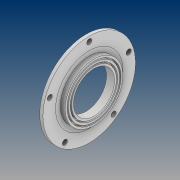
# Autodesk Inventor part: LABYRINTHOSeisodos
Saved by Autodesk Inventor 2021 (Build 250183000, 183)
## iProperties
Created: 2021-01-09
Part Number: LABYRINTHOSeisodos
Material: Generic
Document SubType Name: Modeling
Designer: Διογενης Τσιχλακης
Density: 1 g/cm^3
Appearance: Default
Author: Διογενης Τσιχλακης
Autodesk Inventor part; units mm, degrees
ref_plane "YZ Plane" through (0, 0, 0) normal (1, 0, 0) x (0, 1, 0)
ref_plane "XZ Plane" through (0, 0, 0) normal (0, 1, 0) x (-1, 0, 0)
ref_plane "XY Plane" through (0, 0, 0) normal (0, 0, 1) x (1, 0, 0)
sketch "Sketch1" plane through (0, 0, 0) normal (1, 0, 0) x (0, 1, 0)
  circle A0 centre (0, 0) radius 145
  circle A1 centre (0, 0) radius 115
  circle A2 centre (0, 0) radius 130
  circle A3 centre (130, 0) radius 8
  circle A4 centre (40.1722, 123.6373) radius 8
  circle A5 centre (-105.1722, 76.4121) radius 8
  circle A6 centre (-105.1722, -76.4121) radius 8
  circle A7 centre (40.1722, -123.6373) radius 8
  dimension "d2" = 260
  dimension "d0" = 290
  dimension "d1" = 230
  dimension "d3" = 16
  dimension "d26" = 360
  constraints: 7 centre point, 3 coincident, 1 horizontal alignment, 13 other
  measures "d0" diameter of A0
  measures "d1" diameter of A1
  measures "d3" diameter of A3
extrude "Extrusion1" add sketch "Sketch1" along normal blind 10 contours A0 | A3 A2 A7 A6 A5 A4
sketch "Sketch2" plane through (0, 0, 0) normal (0, 0, 1) x (1, 0, 0)
  line L0 (0, -145) -> (0, 145) projected
  line L1 (0, 115) -> (0, 115.4469)
  line L2 (0, 115.4469) -> (0, 105.4469)
  line L3 (10, -145) -> (10, 145) projected
  line L4 (10, 120.4469) -> (10, 95.4469)
  line L5 (-2, 0) -> (12, 0) projected
  line L6 (0, 105.4469) -> (0, 115)
  line L7 (10, 115) -> (10, -115) projected
  line L8 (10, 115) -> (0, 115)
  line L9 (10, 115) -> (10, 95.4469)
  line L10 (0, 95.4469) -> (0, 105.4469)
  line L11 (0, 95.4469) -> (10, 95.4469)
  point P0 (0, 0)
  constraints: 16 end point, 6 collinear, 3 point on line, 1 perpendicular
revolve "Revolution1" add sketch "Sketch2" angle 360 about axis through (-10, 0, 0) along (1, 0, 0) contours L0 L8 L3 L11
sketch "Sketch3" plane through (0, 0, 0) normal (0, 0, 1) x (1, 0, 0)
  line L0 (15, 90.4469) -> (25, 90.4469)
  line L1 (25, 90.4469) -> (25, 84.4469)
  line L2 (25, 84.4469) -> (15, 84.4469)
  line L3 (10.0111, 105.4469) -> (0, 105.4469)
  line L4 (0, 105.4469) -> (0, 84.4469)
  line L5 (10.0111, 105.4469) -> (0, 105.4469)
  line L6 (15, 84.4469) -> (15, 80.4469)
  line L7 (15, 80.4469) -> (25, 80.4469)
  line L8 (25, 80.4469) -> (25, 75.4469)
  line L9 (25, 75.4469) -> (25, 74.4469)
  line L10 (25, 74.4469) -> (15, 74.4469)
  line L11 (15, 74.4469) -> (15, 70.4469)
  line L12 (15, 70.4469) -> (25, 70.4469)
  line L13 (25, 70.4469) -> (25, 64.4469)
  line L14 (25, 64.4469) -> (0, 64.4469)
  line L15 (0, 64.4469) -> (0, 84.4469)
  line L16 (10.0111, 105.4469) -> (10.0111, 90.4469)
  line L17 (10.0111, 90.4469) -> (15, 90.4469)
  line L18 (-5, 0) -> (30, 0) projected
  point P0 (0, 0)
  constraints: 37 end point, 10 perpendicular, 2 point on line, 1 vertical
revolve "Revolution2" add sketch "Sketch3" angle 360 about axis through (-10, 0, 0) along (1, 0, 0)
thread "Thread7" size "M16x2" class "6H" standard "ANSI Metric M Profile" full length
thread "Thread8" size "M16x2" class "6H" standard "ANSI Metric M Profile" full length
thread "Thread9" size "M16x2" class "6H" standard "ANSI Metric M Profile" full length
thread "Thread10" size "M16x2" class "6H" standard "ANSI Metric M Profile" full length
thread "Thread11" size "M16x2" class "6H" standard "ANSI Metric M Profile" full length
body "Solid1"
